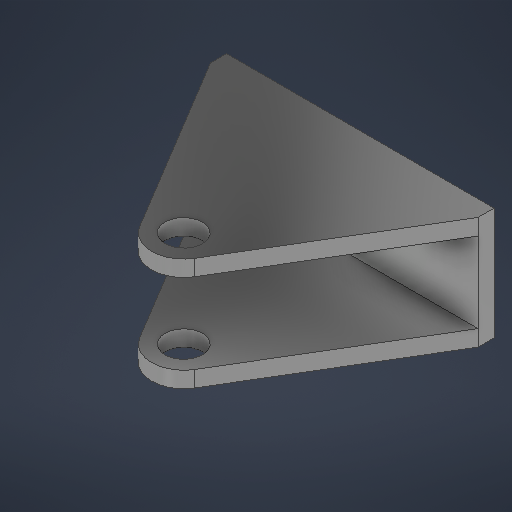
# Autodesk Inventor part: ShifterBracket
Saved by Autodesk Inventor 2026.2 (Build 302298010, 298A)
## iProperties
Created: 2026-07-07
Part Number: ShifterBracket
Material: Generic
Document SubType Name: Modeling
Designer: tasle
Density: 1 g/cm^3
Appearance: Chrome - Polished Black
Author: tasle
Autodesk Inventor part; units mm, degrees
ref_plane "YZ Plane" through (0, 0, 0) normal (1, 0, 0) x (0, 1, 0)
ref_plane "XZ Plane" through (0, 0, 0) normal (0, 1, 0) x (-1, 0, 0)
ref_plane "XY Plane" through (0, 0, 0) normal (0, 0, 1) x (1, 0, 0)
sketch "Sketch1" plane through (0, 0, 0) normal (0, 1, 0) x (-1, 0, 0)
  circle A0 centre (0, 0) radius 3.5
  circle A1 centre (0, 0) radius 6
  line L0 (0, 0) -> (0, -30)
  line L1 (25, -30) -> (-25, -30)
  line L2 (25, -30) -> (5.1448, 3.0873)
  line L3 (-25, -30) -> (-5.1448, 3.0873)
  line L4 (25, -30) -> (-25, -30)
  line L5 (-25, -30) -> (-25, -33)
  line L6 (-25, -33) -> (25, -33)
  line L7 (25, -33) -> (25, -30)
  point P0 (-25, -30)
  dimension "d0" = 7
  dimension "d1" = 12
  dimension "d2" = 30
  dimension "d3" = 50
  dimension "d4" = 3
  constraints: 16 end point, 2 centre point, 2 coincident, 2 horizontal, 2 parallel, 2 point on circle, 2 tangent, 1 midpoint, 1 perpendicular, 1 vertical
  measures "d0" diameter of A0
  measures "d1" diameter of A1
  measures "d2" distance of L0.start L0.end
  measures "d3" distance of L1.start L1.end
  measures "d4" distance of L5.end L4.end
extrude "Extrusion1" add sketch "Sketch1" along normal blind 21
sketch "Sketch2" plane through (0, 0, 0) normal (1, 0, 0) x (0, 1, 0)
  line L0 (18, -30) -> (3, -30)
  line L1 (3, -30) -> (3, 27.9628)
  line L2 (3, 27.9628) -> (18, 27.9628)
  line L3 (18, 27.9628) -> (18, -30)
  line L4 (0, -30) -> (21, -30) projected
  point P0 (0, 0)
  point P1 (10.5, -30)
  dimension "d7" = 15
  constraints: 8 end point, 2 midpoint, 2 parallel, 1 horizontal, 1 perpendicular
  measures "d7" distance of L1.end L2.end
extrude "Extrusion2" cut sketch "Sketch2" along normal mid plane 100
body "Solid1"
